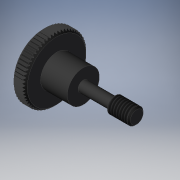
# Autodesk Inventor part: NKOSD3-10
Saved by Autodesk Inventor 2019 (Build 230136000, 136)
## iProperties
Created: 2024-04-23
Part Number: NKOSD3-10
Material: Generic
Catalog Web Link: www.cadenas.de
Description: NOBD, NOOSD, NKBD, NKOSD-Drop-Proof Knurled Knobs
Vendor: MISUMI
Document SubType Name: Modeling
Designer: psAdmin
Manufacturer: MISUMI
Mass: 0.451962 g
Surface Area: 4.93437 cm^2
Volume: 0.451962 cm^3
Density: 1 g/cm^3
Appearance: PSOLRGB-175-175-175
Category: PARTsolutions
Company: MISUMI
Title: NKOSD3-10
Author: Cadenas PARTsolutions
Comments: Drop-Proof Knurled Knobs
PSOL_IDENT_0: {$CADENAS_DATA/23d-libs/misumi/metric/43_levers_knobs/nobd.prj},187 {VTYP=3D},{NB=NKOSD3-10},{LINA=N
PSOL_IDENT_1: KOSD3-10},{NN=NOBD, NOOSD, NKBD, NKOSD},{DATE=04.06.2021 08:39:13},{GEOMDATE=07.02.2014 00:00:00},{V
PSOL_IDENT_2: ERSION=},{LINEID=10},{WBVAR=TS,MAT,LS},{WBNUMERIC=LS}  {NB=NKOSD3-10},{LINA=NKOSD3-10},{KT=DUMMY},{P
PSOL_IDENT_3: N=NKOSD3-10},{TYPE=NKOSD},{TS=2},{MAT=S},{ST=Buffing + Hairline},{M=3},{LS=10},{D=12},{DD=6},{A=2.5}
PSOL_IDENT_4: ,{H=7.5},{S=5.0},{LL=6},{DD2=2.0},{LS1=10},{TIFF=2}
NB: NKOSD3-10
NN: NOBD, NOOSD, NKBD, NKOSD
NT: Drop-Proof Knurled Knobs
NBSYN: $PN.
LINA: NKOSD3-10
CATALOG: Misumi
PN: NKOSD3-10
TS: Threaded with Boss
MAT: 303 Stainless Steel
ST: Buffing + Hairline
M: 3
LS: 10
D: 12
DD: 6
A: 2.5
H: 7.5
S: 5
LL: 6
DD2: 2
SUPPLIER: MISUMI
ARTICLENO: NKOSD3-10
BOMINFO: NKOSD3-10
CREATOR: CADENAS GmbH
Autodesk Inventor part; units mm, degrees
ref_plane "YZ Plane" through (0, 0, 0) normal (1, 0, 0) x (0, 1, 0)
ref_plane "XZ Plane" through (0, 0, 0) normal (0, 1, 0) x (-1, 0, 0)
ref_plane "XY Plane" through (0, 0, 0) normal (0, 0, 1) x (1, 0, 0)
sketch "Sketch_9" plane through (0, 0, 0) normal (0, 0, 1) x (1, 0, 0)
  line L0 (0, 0) -> (-2.5, 0)
  line L1 (-2.5, 0) -> (-2.5, 5.5)
  line L2 (-2.5, 5.5) -> (-2, 6)
  line L3 (-2, 6) -> (-0.5, 6)
  line L4 (-0.5, 6) -> (0, 5.5)
  line L5 (0, 5.5) -> (0, 0)
  line L6 (0, 0) -> (-2.5, 0)
  constraints: 14 end point
revolve "Revolution1" add sketch "Sketch_9" angle 360 about axis through (0, 0, 0) along (1, 0, 0)
sketch "Sketch_3" plane through (0, 0, 0) normal (0, 0, 1) x (1, 0, 0)
  line L0 (5, 0) -> (0, 0)
  line L1 (0, 0) -> (0, 3)
  line L2 (0, 3) -> (5, 3)
  line L3 (5, 3) -> (5, 0)
  line L4 (5, 0) -> (0, 0)
  constraints: 10 end point
revolve "Revolution2" add sketch "Sketch_3" angle 360 about axis through (5, 0, 0) along (1, 0, 0)
sketch "Sketch_4" plane through (0, 0, 0) normal (0, 0, 1) x (1, 0, 0)
  line L0 (15, 0) -> (5, 0)
  line L1 (5, 0) -> (5, 1)
  line L2 (5, 1) -> (11, 1)
  line L3 (11, 1) -> (11, 1.5)
  line L4 (11, 1.5) -> (14.6935, 1.5)
  line L5 (14.6935, 1.5) -> (15, 1.1935)
  line L6 (15, 1.1935) -> (15, 0)
  line L7 (15, 0) -> (5, 0)
  constraints: 16 end point
revolve "Revolution3" add sketch "Sketch_4" angle 360 about axis through (15, 0, 0) along (1, 0, 0)
thread "Thread1" size "M3x0.5" class "6g" standard "ISO Metric profile" full length
sketch "Sketch_1" plane through (0, 0, 0) normal (1, 0, 0) x (0, 1, 0)
  line L0 (-12, 12) -> (-12, -12)
  line L1 (-12, -12) -> (12, -12)
  line L2 (12, -12) -> (12, 12)
  line L3 (12, 12) -> (-12, 12)
  line L4 (0, 6) -> (-0.2983, 5.6922)
  line L5 (-0.2983, 5.6922) -> (-0.6272, 5.9671)
  line L6 (-0.6272, 5.9671) -> (-0.8917, 5.6298)
  line L7 (-0.8917, 5.6298) -> (-1.2475, 5.8689)
  line L8 (-1.2475, 5.8689) -> (-1.4753, 5.5058)
  line L9 (-1.4753, 5.5058) -> (-1.8541, 5.7063)
  line L10 (-1.8541, 5.7063) -> (-2.0427, 5.3214)
  line L11 (-2.0427, 5.3214) -> (-2.4404, 5.4813)
  line L12 (-2.4404, 5.4813) -> (-2.5877, 5.0787)
  line L13 (-2.5877, 5.0787) -> (-3, 5.1962)
  line L14 (-3, 5.1962) -> (-3.1044, 4.7804)
  line L15 (-3.1044, 4.7804) -> (-3.5267, 4.8541)
  line L16 (-3.5267, 4.8541) -> (-3.5871, 4.4297)
  line L17 (-3.5871, 4.4297) -> (-4.0148, 4.4589)
  line L18 (-4.0148, 4.4589) -> (-4.0305, 4.0305)
  line L19 (-4.0305, 4.0305) -> (-4.4589, 4.0148)
  line L20 (-4.4589, 4.0148) -> (-4.4297, 3.5871)
  line L21 (-4.4297, 3.5871) -> (-4.8541, 3.5267)
  line L22 (-4.8541, 3.5267) -> (-4.7804, 3.1044)
  line L23 (-4.7804, 3.1044) -> (-5.1962, 3)
  line L24 (-5.1962, 3) -> (-5.0787, 2.5877)
  line L25 (-5.0787, 2.5877) -> (-5.4813, 2.4404)
  line L26 (-5.4813, 2.4404) -> (-5.3214, 2.0427)
  line L27 (-5.3214, 2.0427) -> (-5.7063, 1.8541)
  line L28 (-5.7063, 1.8541) -> (-5.5058, 1.4753)
  line L29 (-5.5058, 1.4753) -> (-5.8689, 1.2475)
  line L30 (-5.8689, 1.2475) -> (-5.6298, 0.8917)
  line L31 (-5.6298, 0.8917) -> (-5.9671, 0.6272)
  line L32 (-5.9671, 0.6272) -> (-5.6922, 0.2983)
  line L33 (-5.6922, 0.2983) -> (-6, 0)
  line L34 (-6, 0) -> (-5.6922, -0.2983)
  line L35 (-5.6922, -0.2983) -> (-5.9671, -0.6272)
  line L36 (-5.9671, -0.6272) -> (-5.6298, -0.8917)
  line L37 (-5.6298, -0.8917) -> (-5.8689, -1.2475)
  line L38 (-5.8689, -1.2475) -> (-5.5058, -1.4753)
  line L39 (-5.5058, -1.4753) -> (-5.7063, -1.8541)
  line L40 (-5.7063, -1.8541) -> (-5.3214, -2.0427)
  line L41 (-5.3214, -2.0427) -> (-5.4813, -2.4404)
  line L42 (-5.4813, -2.4404) -> (-5.0787, -2.5877)
  line L43 (-5.0787, -2.5877) -> (-5.1962, -3)
  line L44 (-5.1962, -3) -> (-4.7804, -3.1044)
  line L45 (-4.7804, -3.1044) -> (-4.8541, -3.5267)
  line L46 (-4.8541, -3.5267) -> (-4.4297, -3.5871)
  line L47 (-4.4297, -3.5871) -> (-4.4589, -4.0148)
  line L48 (-4.4589, -4.0148) -> (-4.0305, -4.0305)
  line L49 (-4.0305, -4.0305) -> (-4.0148, -4.4589)
  line L50 (-4.0148, -4.4589) -> (-3.5871, -4.4297)
  line L51 (-3.5871, -4.4297) -> (-3.5267, -4.8541)
  line L52 (-3.5267, -4.8541) -> (-3.1044, -4.7804)
  line L53 (-3.1044, -4.7804) -> (-3, -5.1962)
  line L54 (-3, -5.1962) -> (-2.5877, -5.0787)
  line L55 (-2.5877, -5.0787) -> (-2.4404, -5.4813)
  line L56 (-2.4404, -5.4813) -> (-2.0427, -5.3214)
  line L57 (-2.0427, -5.3214) -> (-1.8541, -5.7063)
  line L58 (-1.8541, -5.7063) -> (-1.4753, -5.5058)
  line L59 (-1.4753, -5.5058) -> (-1.2475, -5.8689)
  line L60 (-1.2475, -5.8689) -> (-0.8917, -5.6298)
  line L61 (-0.8917, -5.6298) -> (-0.6272, -5.9671)
  line L62 (-0.6272, -5.9671) -> (-0.2983, -5.6922)
  line L63 (-0.2983, -5.6922) -> (0, -6)
  line L64 (0, -6) -> (0.2983, -5.6922)
  line L65 (0.2983, -5.6922) -> (0.6272, -5.9671)
  line L66 (0.6272, -5.9671) -> (0.8917, -5.6298)
  line L67 (0.8917, -5.6298) -> (1.2475, -5.8689)
  line L68 (1.2475, -5.8689) -> (1.4753, -5.5058)
  line L69 (1.4753, -5.5058) -> (1.8541, -5.7063)
  line L70 (1.8541, -5.7063) -> (2.0427, -5.3214)
  line L71 (2.0427, -5.3214) -> (2.4404, -5.4813)
  line L72 (2.4404, -5.4813) -> (2.5877, -5.0787)
  line L73 (2.5877, -5.0787) -> (3, -5.1962)
  line L74 (3, -5.1962) -> (3.1044, -4.7804)
  line L75 (3.1044, -4.7804) -> (3.5267, -4.8541)
  line L76 (3.5267, -4.8541) -> (3.5871, -4.4297)
  line L77 (3.5871, -4.4297) -> (4.0148, -4.4589)
  line L78 (4.0148, -4.4589) -> (4.0305, -4.0305)
  line L79 (4.0305, -4.0305) -> (4.4589, -4.0148)
  line L80 (4.4589, -4.0148) -> (4.4297, -3.5871)
  line L81 (4.4297, -3.5871) -> (4.8541, -3.5267)
  line L82 (4.8541, -3.5267) -> (4.7804, -3.1044)
  line L83 (4.7804, -3.1044) -> (5.1962, -3)
  line L84 (5.1962, -3) -> (5.0787, -2.5877)
  line L85 (5.0787, -2.5877) -> (5.4813, -2.4404)
  line L86 (5.4813, -2.4404) -> (5.3214, -2.0427)
  line L87 (5.3214, -2.0427) -> (5.7063, -1.8541)
  line L88 (5.7063, -1.8541) -> (5.5058, -1.4753)
  line L89 (5.5058, -1.4753) -> (5.8689, -1.2475)
  line L90 (5.8689, -1.2475) -> (5.6298, -0.8917)
  line L91 (5.6298, -0.8917) -> (5.9671, -0.6272)
  line L92 (5.9671, -0.6272) -> (5.6922, -0.2983)
  line L93 (5.6922, -0.2983) -> (6, 0)
  line L94 (6, 0) -> (5.6922, 0.2983)
  line L95 (5.6922, 0.2983) -> (5.9671, 0.6272)
  line L96 (5.9671, 0.6272) -> (5.6298, 0.8917)
  line L97 (5.6298, 0.8917) -> (5.8689, 1.2475)
  line L98 (5.8689, 1.2475) -> (5.5058, 1.4753)
  line L99 (5.5058, 1.4753) -> (5.7063, 1.8541)
  line L100 (5.7063, 1.8541) -> (5.3214, 2.0427)
  line L101 (5.3214, 2.0427) -> (5.4813, 2.4404)
  line L102 (5.4813, 2.4404) -> (5.0787, 2.5877)
  line L103 (5.0787, 2.5877) -> (5.1962, 3)
  line L104 (5.1962, 3) -> (4.7804, 3.1044)
  line L105 (4.7804, 3.1044) -> (4.8541, 3.5267)
  line L106 (4.8541, 3.5267) -> (4.4297, 3.5871)
  line L107 (4.4297, 3.5871) -> (4.4589, 4.0148)
  line L108 (4.4589, 4.0148) -> (4.0305, 4.0305)
  line L109 (4.0305, 4.0305) -> (4.0148, 4.4589)
  line L110 (4.0148, 4.4589) -> (3.5871, 4.4297)
  line L111 (3.5871, 4.4297) -> (3.5267, 4.8541)
  line L112 (3.5267, 4.8541) -> (3.1044, 4.7804)
  line L113 (3.1044, 4.7804) -> (3, 5.1962)
  line L114 (3, 5.1962) -> (2.5877, 5.0787)
  line L115 (2.5877, 5.0787) -> (2.4404, 5.4813)
  line L116 (2.4404, 5.4813) -> (2.0427, 5.3214)
  line L117 (2.0427, 5.3214) -> (1.8541, 5.7063)
  line L118 (1.8541, 5.7063) -> (1.4753, 5.5058)
  line L119 (1.4753, 5.5058) -> (1.2475, 5.8689)
  line L120 (1.2475, 5.8689) -> (0.8917, 5.6298)
  line L121 (0.8917, 5.6298) -> (0.6272, 5.9671)
  line L122 (0.6272, 5.9671) -> (0.2983, 5.6922)
  line L123 (0.2983, 5.6922) -> (0, 6)
  constraints: 248 end point
extrude "Extrusion1" cut sketch "Sketch_1" against normal blind 2.5
body "Solid1"
